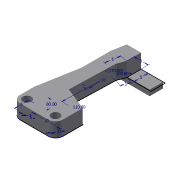
# Autodesk Inventor part: gripper
Saved by Autodesk Inventor 2018 (Build 220112000, 112)
## iProperties
Created: 2018-08-17
Part Number: gripper
Material: Generic
Document SubType Name: Modeling
Designer: Bardo91
Density: 1 g/cm^3
Appearance: Default
Author: Bardo91
Autodesk Inventor part; units mm, degrees
ref_plane "YZ Plane" through (0, 0, 0) normal (1, 0, 0) x (0, 1, 0)
ref_plane "XZ Plane" through (0, 0, 0) normal (0, 1, 0) x (-1, 0, 0)
ref_plane "XY Plane" through (0, 0, 0) normal (0, 0, 1) x (1, 0, 0)
sketch "Sketch1" plane through (0, 0, 0) normal (0, 0, 1) x (1, 0, 0)
  line L0 (0, 0) -> (10, 0)
  circle A0 centre (0, 0) radius 1.5
  circle A1 centre (10, 0) radius 1.5
  circle A2 centre (0, 0) radius 2.5
  circle A3 centre (10, 0) radius 2.5
  line L1 (0, -2.5) -> (10, -2.5)
  line L2 (-2.5, 0) -> (-2.5, 5)
  line L3 (-2.5, 5) -> (0, 19.1782)
  line L4 (-2.5, 5) -> (11.8969, 5) construction
  line L5 (0, 19.1782) -> (0, 29.1782)
  line L6 (0, 29.1782) -> (0.8682, 34.1022)
  line L7 (0.8682, 34.1022) -> (5.8682, 34.1022)
  line L8 (5.8682, 34.1022) -> (5.8682, 29.1022)
  line L9 (5.8682, 29.1022) -> (4.8422, 26.2832)
  line L10 (4.8422, 26.2832) -> (4.3644, 10.2903)
  line L11 (4.3644, 10.2903) -> (12.5, 7.0509)
  line L12 (12.5, 7.0509) -> (12.5, 0)
  line L13 (5.8682, 34.1022) -> (14.2847, 34.1022)
  line L14 (14.2847, 34.1022) -> (14.2847, 29.1022)
  line L15 (14.2847, 29.1022) -> (5.8682, 29.1022)
  dimension "d0" = 10
  dimension "d1" = 3
  dimension "d2" = 3
  dimension "d3" = 5
  dimension "d4" = 5
  dimension "d5" = 5
  dimension "d6" = 80
  dimension "d7" = 10
  dimension "d8" = 5
  dimension "d9" = 170
  dimension "d10" = 5
  dimension "d11" = 5
  dimension "d12" = 3
  dimension "d13" = 160
  dimension "d14" = 16
  dimension "d15" = 110
  constraints: 32 end point, 5 perpendicular, 4 centre point, 4 coincident, 4 horizontal, 4 point on circle, 2 parallel, 1 equal length, 1 vertical
  measures "d0" distance of L0.start L0.end
  measures "d1" diameter of A0
  measures "d2" diameter of A1
  measures "d3" diameter of A2
  measures "d4" diameter of A3
  measures "d5" distance of L2.start L2.end
  measures "d6" angle of L4 L3
  measures "d7" distance of L3.end L5.end
  measures "d8" distance of L5.end L6.end
  measures "d9" angle of L5 L6
  measures "d10" distance of L6.end L7.end
  measures "d11" distance of L7.end L8.end
  measures "d12" distance of L8.end L9.end
  measures "d13" angle of L8 L9
  measures "d14" distance of L9.end L10.end
  measures "d15" angle of L11 L10
extrude "Extrusion1" add sketch "Sketch1" along normal blind 5 contours A2 | A2 L2 L3 L5 L6 L7 L8 L9 L10 L11 L12 A3 L0 | L0 A3 L1 A2 | A3
sketch "Sketch2" plane through (0, 0, 0) normal (0, 0, -1) x (-1, 0, 0)
  line L0 (-5.8682, 34.1022) -> (-0.8682, 34.1022) projected
  line L1 (-0.8682, 34.1022) -> (-13.6111, 34.1022)
  line L2 (-13.6111, 34.1022) -> (-13.6111, 29.3872)
  line L3 (-13.6111, 29.3872) -> (-0.8682, 29.3872)
  line L4 (-0.8682, 29.3872) -> (-0.8682, 34.1022)
  point P0 (0, 0)
  constraints: 8 end point, 2 parallel, 1 horizontal, 1 perpendicular
extrude "Extrusion3" add sketch "Sketch2" along normal blind 2
body "Solid1"
